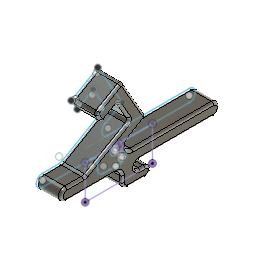
ID.3 Anchor (Autodesk Fusion 360 design; units mm, degrees)
part number: 2026-06-05-21-03-36-349
Autodesk Fusion 360 part; units mm, degrees
sketch "Sample car slot" plane through (0, 0, 0) normal (0, 0, 1) x (1, 0, 0)
  line L0 (0, 0) -> (-30, 0)
  line L1 (-30, 0) -> (-30, 55)
  line L2 (-30, 55) -> (0, 55)
  line L3 (0, 55) -> (0, 0)
  line L4 (-35, -5) -> (-35, 60)
  line L5 (-35, 60) -> (5, 60)
  line L6 (5, 60) -> (5, -5)
  line L7 (5, -5) -> (-35, -5)
  line L8 (-30, 24.5) -> (0, 24.5)
  line L9 (-30, 30.5) -> (0, 30.5)
  dimension "d10" = 30
  dimension "d11" = 55
  dimension "d17" = -5
  dimension "d27" = 6
  constraint horizontal L0
  constraint vertical L1
  constraint horizontal L2
  constraint vertical L3
  constraint coincident L0.start L3.end
  measures "d10" distance of L0.start L0.end
  measures "d11" distance of L0.start L2.end
  measures "d27" distance of L8 L9
extrude "Extrude2" add sketch "Sample car slot" against normal blind 30 contours L0 L1 L3 L8 | L1 L3 L8 L9 | L1 L2 L3 L9 | L4 L5 L6 L7 makes body 1
extrude "Extrude3" cut sketch "Sample car slot" against normal blind 28 contours L0 L1 L3 L8 | L1 L3 L8 L9 | L1 L2 L3 L9 bodies 1
sketch "Sample anchor bar" plane through (-35, 0, 0) normal (-1, 0, 0) x (0, -1, 0)
  line L0 (5, 0) -> (-60, 0)
  line L1 (-60, 0) -> (-60, -30)
  line L2 (-60, -30) -> (5, -30)
  line L3 (5, -30) -> (5, 0)
  circle A0 centre (-27.5, -3) radius 3
  dimension "d28" = 32.5
  measures "d28" distance of L3 A0.centre
extrude "Extrude5" add sketch "Sample anchor bar" against normal up to surface (35 mm away) contours A0 bodies 1
sketch "Anchor type 1" plane through (-30, 0, 0) normal (1, 0, 0) x (0, 1, 0)
  line L0 (27.5, 0) -> (0, 0)
  line L1 (0, 0) -> (0, -28)
  line L2 (0, -28) -> (55, -28)
  line L3 (55, -28) -> (55, 0)
  line L4 (55, 0) -> (27.5, 0)
  circle A0 centre (27.5, -3) radius 3
  line L5 (24.6702, -22.5732) -> (24.6702, -16.6727)
  line L6 (30.3298, -22.5732) -> (30.3298, -16.6727)
  arc A1 (32.809, -24.515) -> (49.6413, -2.0828) centre (27.5, -3) ccw
  arc A2 (31.6637, -14.7869) -> (39.9438, -1.8095) centre (27.5, -3) ccw
  arc A3 (15.0562, -1.8095) -> (23.3363, -14.7869) centre (27.5, -3) ccw
  arc A4 (5.3587, -2.0828) -> (22.191, -24.515) centre (27.5, -3) ccw
  line L7 (80, 2) -> (80, 3)
  line L8 (-25, 3) -> (-25, 2)
  line L9 (-23, 0) -> (3.3604, 0)
  line L10 (17.0471, 0) -> (37.9529, 0)
  line L11 (51.6396, 0) -> (78, 0)
  line L12 (37.0885, 5.5359) -> (67.3372, 23)
  line L13 (27.5, 0) -> (57.5, 0) construction
  line L14 (68.8013, 28.4641) -> (57.8013, 47.5167)
  line L15 (70.8013, 25) -> (73.4808, 25) construction
  line L16 (52.3372, 48.9808) -> (46.275, 45.4808)
  line L17 (82.4615, 24.8038) -> (61.4615, 61.1769)
  line L18 (55.9974, 62.641) -> (41.275, 54.141)
  line L19 (39.8109, 48.6769) -> (40.8109, 46.9449)
  line L20 (69.0885, 12.4641) -> (80.9974, 19.3397)
  line L21 (78, 5) -> (71.0885, 5)
  line L22 (35.0885, 5) -> (-23, 5)
  line L23 (27.5, -3) -> (27.5, -6)
  arc A5 (69.0885, 12.4641) -> (71.0885, 5) centre (71.0885, 9) ccw
  arc A6 (80.9974, 19.3397) -> (82.4615, 24.8038) centre (78.9974, 22.8038) ccw
  arc A7 (67.3372, 23) -> (68.8013, 28.4641) centre (65.3372, 26.4641) ccw
  arc A8 (57.8013, 47.5167) -> (52.3372, 48.9808) centre (54.3372, 45.5167) ccw
  arc A9 (61.4615, 61.1769) -> (55.9974, 62.641) centre (57.9974, 59.1769) ccw
  arc A10 (41.275, 54.141) -> (39.8109, 48.6769) centre (43.275, 50.6769) ccw
  arc A11 (40.8109, 46.9449) -> (46.275, 45.4808) centre (44.275, 48.9449) ccw
  arc A12 (35.0885, 5) -> (37.0885, 5.5359) centre (35.0885, 9) ccw
  arc A13 (78, 0) -> (80, 2) centre (78, 2) ccw
  arc A14 (80, 3) -> (78, 5) centre (78, 3) ccw
  arc A15 (-23, 5) -> (-25, 3) centre (-23, 3) ccw
  arc A16 (-25, 2) -> (-23, 0) centre (-23, 2) ccw
  arc A17 (39.9438, -1.8095) -> (37.9529, 0) centre (37.9529, -2) ccw
  arc A18 (51.6396, 0) -> (49.6413, -2.0828) centre (51.6396, -2) ccw
  arc A19 (17.0471, 0) -> (15.0562, -1.8095) centre (17.0471, -2) ccw
  arc A20 (5.3587, -2.0828) -> (3.3604, 0) centre (3.3604, -2) ccw
  arc A21 (24.6702, -16.6727) -> (23.3363, -14.7869) centre (22.6702, -16.6727) ccw
  arc A22 (22.191, -24.515) -> (24.6702, -22.5732) centre (22.6702, -22.5732) ccw
  arc A23 (30.3298, -22.5732) -> (32.809, -24.515) centre (32.3298, -22.5732) ccw
  arc A24 (31.6637, -14.7869) -> (30.3298, -16.6727) centre (32.3298, -16.6727) ccw
  point P0 (55.8013, 50.9808)
  point P1 (42.8109, 43.4808)
  dimension "d32" = 30
  dimension "d33" = 50
  dimension "d34" = 120
  dimension "d35" = 30
  dimension "d36" = 15
  dimension "d38" = 4
  dimension "d39" = 4
  dimension "d40" = 2
  dimension "d41" = 2
  dimension "d42" = 2
  constraint coincident A0.centre A1.centre
  constraint horizontal L9
  constraint vertical L7
  constraint horizontal L21
  constraint vertical L8
  constraint collinear L9 L10
  constraint collinear L10 L11
  constraint horizontal L13
  constraint coincident L0.start L4.end
  constraint horizontal L15
  constraint perpendicular L14 L16
  constraint perpendicular L16 L19
  constraint collinear L21 L22
  constraint coincident A0 L23.end
  constraint tangent L21 A5
  constraint tangent L20 A5
  constraint tangent L20 A6
  constraint tangent L17 A6
  constraint coincident L15.start L12
  constraint coincident L15.start L14
  constraint tangent L12 A7
  constraint tangent L14 A7
  constraint equal A6 A7
  constraint coincident P0 L14
  constraint coincident P0 L16
  constraint tangent L14 A8
  constraint tangent L16 A8
  constraint equal A6 A8
  constraint tangent L17 A9
  constraint tangent L18 A9
  constraint equal A6 A9
  constraint tangent L18 A10
  constraint tangent L19 A10
  constraint equal A6 A10
  constraint coincident P1 L16
  constraint coincident P1 L19
  constraint tangent L16 A11
  constraint tangent L19 A11
  constraint equal A6 A11
  constraint tangent L12 A12
  constraint tangent L22 A12
  constraint equal A6 A12
  constraint tangent L7 A13
  constraint tangent L11 A13
  constraint tangent L7 A14
  constraint tangent L21 A14
  constraint equal A13 A14
  constraint tangent L8 A15
  constraint tangent L22 A15
  constraint equal A13 A15
  constraint tangent L8 A16
  constraint tangent L9 A16
  constraint equal A13 A16
  constraint tangent A2 A17
  constraint tangent L10 A17
  constraint equal A13 A17
  constraint tangent A1 A18
  constraint tangent L11 A18
  constraint equal A13 A18
  constraint tangent A3 A19
  constraint tangent L10 A19
  constraint equal A13 A19
  constraint tangent A4 A20
  constraint tangent L9 A20
  constraint equal A13 A20
  constraint tangent A3 A21
  constraint tangent L5 A21
  constraint tangent A4 A22
  constraint tangent L5 A22
  constraint tangent L6 A23
  constraint tangent A1 A23
  constraint equal A22 A23
  constraint tangent A2 A24
  constraint tangent L6 A24
  constraint equal A22 A24
  measures "d32" angle of L12 L13
  measures "d33" distance of L0.start L15.start
  measures "d34" angle of L14 L15
  measures "d35" distance of L15.start P0
  measures "d36" distance of P0 P1
  measures "d38" radius of A5
  measures "d39" radius of A6
  measures "d40" radius of A13
  measures "d41" radius of A21
  measures "d42" radius of A22
extrude "Extrude6" add sketch "Anchor type 1" along normal blind 20 separate body contours L0 L4 L7 L8 L9 L10 L11 L12 L14 L16 L17 L18 L19 L20 L21 L22 A5 A6 A7 A8 A9 A10 A11 A12 A13 A14 A15 A16 | L0 L5 A3 A4 A19 A20 A21 A22 | L4 L6 A1 A2 A17 A18 A23 A24 makes body 2
sketch "Anchor type 2" plane through (-30, 0, 0) normal (1, 0, 0) x (0, 1, 0)
  line L0 (27.5, 0) -> (0, 0)
  line L1 (0, 0) -> (0, -28)
  line L2 (0, -28) -> (55, -28)
  line L3 (55, -28) -> (55, 0)
  line L4 (55, 0) -> (27.5, 0)
  circle A0 centre (27.5, -3) radius 3
  line L5 (25, -7) -> (29, -7)
  line L6 (20, -15) -> (15, -15)
  line L7 (10, -10) -> (10, -5)
  line L8 (85, 0) -> (25, 0)
  line L9 (5, 0) -> (-35, 0)
  line L10 (16.1603, 19.3301) -> (28.1458, 26.25)
  line L11 (0, 10) -> (35, 10) construction
  line L12 (29.0609, 29.6651) -> (20.3109, 44.8205)
  line L13 (14.4856, 29.9103) -> (-18.8397, 10.6699)
  line L14 (20.3109, 44.8205) -> (11.5609, 59.976)
  line L15 (8.1458, 60.891) -> (1.6506, 57.141)
  line L16 (4.4856, 47.2308) -> (-4.1747, 42.2308)
  line L17 (-7.5897, 43.1458) -> (-10.0897, 47.476)
  line L18 (-9.1747, 50.891) -> (1.6506, 57.141)
  line L19 (7.9006, 46.3157) -> (15.4006, 33.3253)
  line L20 (-35, 10) -> (-21.3397, 10)
  line L21 (18.6603, 10) -> (85, 10)
  arc A1 (-9.1747, 50.891) -> (-10.0897, 47.476) centre (-7.9247, 48.726) ccw
  arc A2 (-7.5897, 43.1458) -> (-4.1747, 42.2308) centre (-5.4247, 44.3958) ccw
  arc A3 (7.9006, 46.3157) -> (4.4856, 47.2308) centre (5.7356, 45.0657) ccw
  arc A4 (14.4856, 29.9103) -> (15.4006, 33.3253) centre (13.2356, 32.0753) ccw
  arc A5 (11.5609, 59.976) -> (8.1458, 60.891) centre (9.3958, 58.726) ccw
  arc A6 (28.1458, 26.25) -> (29.0609, 29.6651) centre (26.8958, 28.4151) ccw
  arc A7 (16.1603, 19.3301) -> (18.6603, 10) centre (18.6603, 15) ccw
  arc A8 (-21.3397, 10) -> (-18.8397, 10.6699) centre (-21.3397, 15) ccw
  arc A9 (-35, 10) -> (-40, 5) centre (-35, 5) ccw
  arc A10 (-40, 5) -> (-35, 0) centre (-35, 5) ccw
  arc A11 (85, 0) -> (90, 5) centre (85, 5) ccw
  arc A12 (90, 5) -> (85, 10) centre (85, 5) ccw
  arc A13 (25, 0) -> (21.6928, -1.25) centre (25, -5) ccw
  arc A14 (21.6928, -5.75) -> (25, -7) centre (25, -2) ccw
  arc A15 (10, -5) -> (5, 0) centre (5, -5) ccw
  arc A16 (10, -10) -> (15, -15) centre (15, -10) ccw
  arc A17 (33.3301, -9.5) -> (29, -7) centre (29, -12) ccw
  arc A18 (29, -15) -> (33.3301, -12.5) centre (29, -10) ccw
  arc A19 (21.6928, -1.25) -> (21.6928, -5.75) centre (23.6771, -3.5) ccw
  arc A20 (33.3301, -12.5) -> (33.3301, -9.5) centre (30.7321, -11) ccw
  line L22 (29, -15) -> (25, -15)
  line L23 (25, -15) -> (20, -15)
  point P0 (30.3109, 27.5)
  point P1 (10.3109, 62.141)
  point P2 (6.6506, 48.4808)
  point P3 (-6.3397, 40.9808)
  point P4 (-11.3397, 49.641)
  dimension "d45" = 30
  dimension "d46" = 35
  dimension "d47" = 20
  dimension "d48" = 20
  dimension "d49" = 10
  dimension "d50" = 10
  dimension "d51" = 15
  dimension "d52" = 10
  dimension "d53" = 2.5
  dimension "d54" = 5
  dimension "d55" = 5
  dimension "d56" = 3
  dimension "d57" = 3
  constraint parallel L4 L8
  constraint collinear L8 L9
  constraint horizontal L11
  constraint perpendicular L10 L12
  constraint perpendicular L12 L13
  constraint perpendicular L13 L14
  constraint perpendicular L14 L15
  constraint perpendicular L15 L17
  constraint perpendicular L13 L19
  constraint collinear L20 L21
  constraint coincident P4 L17
  constraint coincident P4 L18
  constraint tangent L17 A1
  constraint tangent L18 A1
  constraint coincident P3 L16
  constraint coincident P3 L17
  constraint tangent L16 A2
  constraint tangent L17 A2
  constraint equal A1 A2
  constraint coincident P2 L16
  constraint coincident P2 L19
  constraint tangent L16 A3
  constraint tangent L19 A3
  constraint equal A1 A3
  constraint tangent L19 A4
  constraint tangent L13 A4
  constraint equal A1 A4
  constraint coincident P1 L14
  constraint coincident P1 L15
  constraint tangent L14 A5
  constraint tangent L15 A5
  constraint equal A1 A5
  constraint coincident P0 L10
  constraint coincident P0 L12
  constraint tangent L10 A6
  constraint tangent L12 A6
  constraint equal A1 A6
  constraint coincident L11.start L10
  constraint coincident L11.start L21
  constraint tangent L10 A7
  constraint tangent L21 A7
  constraint tangent L13 A8
  constraint tangent L20 A8
  constraint tangent L20 A9
  constraint equal A8 A9
  constraint tangent L9 A10
  constraint equal A8 A10
  constraint coincident A9.end A10.start
  constraint tangent L8 A11
  constraint equal A8 A11
  constraint tangent L21 A12
  constraint equal A8 A12
  constraint coincident A11.end A12.start
  constraint tangent L8 A13
  constraint equal A8 A13
  constraint tangent L5 A14
  constraint equal A8 A14
  constraint tangent L7 A15
  constraint tangent L9 A15
  constraint equal A8 A15
  constraint tangent L6 A16
  constraint tangent L7 A16
  constraint equal A8 A16
  constraint tangent L5 A17
  constraint equal A8 A17
  constraint tangent A18 L22
  constraint equal A8 A18
  constraint tangent A14 A19
  constraint tangent A13 A19
  constraint tangent A18 A20
  constraint tangent A17 A20
  measures "d45" angle of L10 L11
  measures "d46" distance of L11.start P0
  measures "d47" distance of P0 L12.end
  measures "d48" distance of L12.end P1
  measures "d49" distance of P1 L15.end
  measures "d50" distance of L15.end P2
  measures "d51" distance of P2 P3
  measures "d52" distance of P3 P4
  measures "d53" radius of A1
  measures "d54" radius of A7
  measures "d55" radius of A8
  measures "d56" radius of A19
  measures "d57" radius of A20
extrude "Extrude7" add sketch "Anchor type 2" along normal blind 20 separate body contours L0 L4 L8 L9 L10 L12 L13 L14 L15 L16 L17 L18 L19 L20 L21 A1 A2 A3 A4 A5 A6 A7 A8 A9 A10 A11 A12 | L0 L5 L6 L7 A13 A14 A15 A16 A17 A18 A19 A20 L22 L23 makes body 3
fillet "Fillet1" radius 2 1 faces at (-10, -1.7258, 8.6051) on bodies 3
fillet "Fillet2" radius 2 1 faces at (-30, -0.0591, 8.6051) on bodies 3
hidden bodies 1 2
equation "d28 = ( 65 / 2 ) * 1 mm"
named bodies: "Sample car slot", "Anchor type 1", "Anchor type 2"
